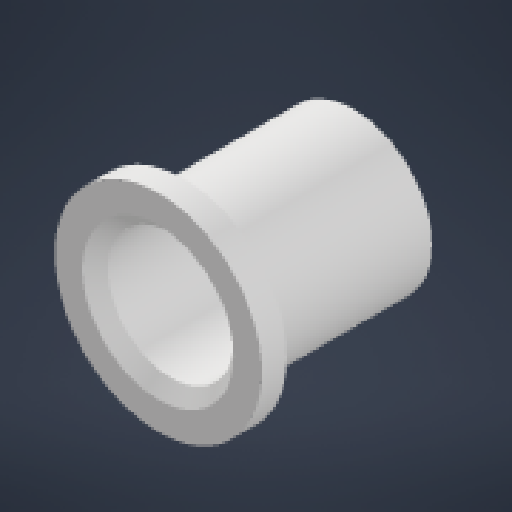
# Autodesk Inventor part: AxleAdapter
Saved by Autodesk Inventor 2024.1 (Build 281209000, 209)
## iProperties
Created: 2023-10-19
Part Number: AxleAdapter
Material: Generic
Document SubType Name: Modeling
Designer: Brandon
Density: 1 g/cm^3
Appearance: Default
Author: Brandon
Autodesk Inventor part; units mm, degrees
ref_plane "YZ Plane" through (0, 0, 0) normal (1, 0, 0) x (0, 1, 0)
ref_plane "XZ Plane" through (0, 0, 0) normal (0, 1, 0) x (-1, 0, 0)
ref_plane "XY Plane" through (0, 0, 0) normal (0, 0, 1) x (1, 0, 0)
sketch "Sketch1" plane through (0, 0, 0) normal (0, 0, 1) x (1, 0, 0)
  circle A0 centre (0, 0) radius 4 projected
  circle A1 centre (0, 0) radius 3.9492
  circle A2 centre (0, 0) radius 5.2192
  circle A3 centre (0, 0) radius 3.175
  point P0 (0, 0)
  dimension "d0" = 0.0508
  dimension "d1" = 1.27
  dimension "d2" = 6.35
  constraints: 3 centre point, 1 coincident
  measures "d0" radial gap between concentric circles of A0 A1
  measures "d1" radial gap between concentric circles of A1 A2
  measures "d2" diameter of A3
extrude "Extrusion1" add sketch "Sketch1" along normal blind 1.27 contours A0 | A1 | A2
extrude "Extrusion2" add sketch "Sketch1" against normal blind 8.5875 contours A1
chamfer "Chamfer1" distance 0.635 angle 45 1 edges at (-3.175, 0, 1.27)
body "Solid1"
